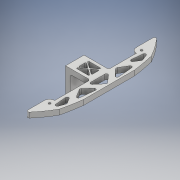
# Autodesk Inventor part: ガイド横v1
Saved by Autodesk Inventor 2018.3 (Build 223284000, 284)
## iProperties
Created: 2019-02-14
Part Number: ガイド横v1
Material: 一般
Document SubType Name: Modeling
Designer: shun2
Density: 1 g/cm^3
Appearance: 既定
Author: shun2
Autodesk Inventor part; units mm, degrees
ref_plane "YZ Plane" through (0, 0, 0) normal (1, 0, 0) x (0, 1, 0)
ref_plane "XZ Plane" through (0, 0, 0) normal (0, 1, 0) x (-1, 0, 0)
ref_plane "XY Plane" through (0, 0, 0) normal (0, 0, 1) x (1, 0, 0)
sketch "スケッチ1" plane through (0, 0, 0) normal (0, 0, 1) x (1, 0, 0)
  circle A0 centre (7, 27.638) radius 1.5
  circle A1 centre (7, 152.362) radius 1.5
  arc A2 (0, 0) -> (20.2574, 27.638) centre (-93.8083, 90) ccw
  arc A3 (20.2574, 152.362) -> (0, 180) centre (-93.8083, 90) ccw
  arc A4 (0, 152.362) -> (7, 145.362) centre (7, 152.362) ccw
  arc A5 (7, 34.638) -> (0, 27.638) centre (7, 27.638) ccw
  line L0 (7, 34.638) -> (7, 145.362)
  line L1 (0, 180) -> (0, 152.362)
  line L2 (0, 27.638) -> (0, 0)
  line L3 (25.3494, 124.4636) -> (25.3494, 55.5364)
  arc A6 (20.2574, 27.638) -> (25.3494, 55.5364) centre (-242.442, 90) ccw
  arc A7 (25.3494, 124.4636) -> (20.2574, 152.362) centre (-242.442, 90) ccw
  point P0 (7, 20.638)
  point P1 (7, 159.362)
  dimension "d2" = 3
  dimension "d11" = 27.638
  constraints: 12 point on circle, 8 centre point, 8 end point, 4 vertical, 2 coincident, 2 point on line
  measures "d2" diameter of A0
  measures "d11" vertical distance of L2.end A0.centre
extrude "押し出し1" add sketch "スケッチ1" along normal blind 7
sketch "スケッチ2" plane through (0, 0, 7) normal (0, 0, 1) x (1, 0, 0)
  line L0 (10, 80.2837) -> (10, 99.7163)
  line L1 (13.4987, 101.0407) -> (22.0846, 91.3243)
  line L2 (22.0846, 88.6757) -> (13.4987, 78.9593)
  line L3 (19.2111, 75.7008) -> (11.0046, 66.6519)
  line L4 (10.7784, 64.2673) -> (17.1291, 53.8503)
  line L5 (20.8277, 54.7016) -> (22.6836, 74.1675)
  line L6 (14.4979, 46.7358) -> (18.8075, 39.7711)
  line L7 (18.979, 38.0154) -> (16.0642, 30.2561)
  line L8 (12.2009, 30.7708) -> (10.8061, 45.4948)
  arc A0 (18.979, 38.0154) -> (18.8075, 39.7711) centre (17.1068, 38.7188) ccw
  arc A1 (11.0046, 66.6519) -> (10.7784, 64.2673) centre (12.4861, 65.3083) ccw
  arc A2 (22.0846, 88.6757) -> (22.0846, 91.3243) centre (20.5859, 90) ccw
  arc A3 (12.2009, 30.7708) -> (16.0642, 30.2561) centre (14.192, 30.9595) ccw
  arc A4 (14.4979, 46.7358) -> (10.8061, 45.4948) centre (12.7972, 45.6834) ccw
  arc A5 (17.1291, 53.8503) -> (20.8277, 54.7016) centre (18.8368, 54.8914) ccw
  arc A6 (22.6836, 74.1675) -> (19.2111, 75.7008) centre (20.6926, 74.3573) ccw
  arc A7 (10, 80.2837) -> (13.4987, 78.9593) centre (12, 80.2837) ccw
  arc A8 (13.4987, 101.0407) -> (10, 99.7163) centre (12, 99.7163) ccw
  line L9 (19.2111, 104.2992) -> (11.0046, 113.3481)
  line L10 (10.7784, 115.7327) -> (17.1291, 126.1497)
  line L11 (20.8277, 125.2984) -> (22.6836, 105.8325)
  line L12 (14.4979, 133.2642) -> (18.8075, 140.2289)
  line L13 (18.979, 141.9846) -> (16.0642, 149.7439)
  line L14 (12.2009, 149.2292) -> (10.8061, 134.5052)
  arc A9 (18.8075, 140.2289) -> (18.979, 141.9846) centre (17.1068, 141.2812) ccw
  arc A10 (10.7784, 115.7327) -> (11.0046, 113.3481) centre (12.4861, 114.6917) ccw
  arc A11 (16.0642, 149.7439) -> (12.2009, 149.2292) centre (14.192, 149.0405) ccw
  arc A12 (10.8061, 134.5052) -> (14.4979, 133.2642) centre (12.7972, 134.3166) ccw
  arc A13 (20.8277, 125.2984) -> (17.1291, 126.1497) centre (18.8368, 125.1086) ccw
  arc A14 (19.2111, 104.2992) -> (22.6836, 105.8325) centre (20.6926, 105.6427) ccw
  point P0 (0, 0)
  point P1 (10, 75)
  point P2 (10, 105)
  dimension "d17" = 30
  dimension "d18" = 2
  constraints: 30 end point, 30 point on circle, 18 tangent, 15 centre point, 8 equal radius, 4 point on line, 1 vertical
  measures "d17" distance of point (10, 75) point (10, 105)
  measures "d18" radius of A0
extrude "押し出し2" cut sketch "スケッチ2" against normal blind 7
fillet "フィレット1" radius 2 2 edges at (0, 180, 3.5) (0, 0, 3.5)
sketch "スケッチ3" plane through (0, 0, 7) normal (0, 0, 1) x (1, 0, 0)
  arc A0 (20.8277, 125.2984) -> (17.1291, 126.1497) centre (18.8368, 125.1086) ccw projected
  line L0 (17.1291, 126.1497) -> (10.7784, 115.7327) projected
  arc A1 (10.7784, 115.7327) -> (11.0046, 113.3481) centre (12.4861, 114.6917) ccw projected
  line L1 (11.0046, 113.3481) -> (19.2111, 104.2992) projected
  arc A2 (19.2111, 104.2992) -> (22.6836, 105.8325) centre (20.6926, 105.6427) ccw projected
  line L2 (22.6836, 105.8325) -> (20.8277, 125.2984) projected
  arc A3 (18.8075, 140.2289) -> (18.979, 141.9846) centre (17.1068, 141.2812) ccw projected
  line L3 (18.979, 141.9846) -> (16.0642, 149.7439) projected
  arc A4 (16.0642, 149.7439) -> (12.2009, 149.2292) centre (14.192, 149.0405) ccw projected
  line L4 (12.2009, 149.2292) -> (10.8061, 134.5052) projected
  arc A5 (10.8061, 134.5052) -> (14.4979, 133.2642) centre (12.7972, 134.3166) ccw projected
  line L5 (14.4979, 133.2642) -> (18.8075, 140.2289) projected
  arc A6 (14.4979, 46.7358) -> (10.8061, 45.4948) centre (12.7972, 45.6834) ccw projected
  line L6 (10.8061, 45.4948) -> (12.2009, 30.7708) projected
  arc A7 (12.2009, 30.7708) -> (16.0642, 30.2561) centre (14.192, 30.9595) ccw projected
  line L7 (16.0642, 30.2561) -> (18.979, 38.0154) projected
  arc A8 (18.979, 38.0154) -> (18.8075, 39.7711) centre (17.1068, 38.7188) ccw projected
  line L8 (18.8075, 39.7711) -> (14.4979, 46.7358) projected
  arc A9 (11.0046, 66.6519) -> (10.7784, 64.2673) centre (12.4861, 65.3083) ccw projected
  line L9 (10.7784, 64.2673) -> (17.1291, 53.8503) projected
  arc A10 (17.1291, 53.8503) -> (20.8277, 54.7016) centre (18.8368, 54.8914) ccw projected
  line L10 (20.8277, 54.7016) -> (22.6836, 74.1675) projected
  arc A11 (22.6836, 74.1675) -> (19.2111, 75.7008) centre (20.6926, 74.3573) ccw projected
  line L11 (19.2111, 75.7008) -> (11.0046, 66.6519) projected
  arc A12 (13.4987, 101.0407) -> (10, 99.7163) centre (12, 99.7163) ccw projected
  line L12 (10, 99.7163) -> (10, 80.2837) projected
  arc A13 (10, 80.2837) -> (13.4987, 78.9593) centre (12, 80.2837) ccw projected
  line L13 (13.4987, 78.9593) -> (22.0846, 88.6757) projected
  arc A14 (22.0846, 88.6757) -> (22.0846, 91.3243) centre (20.5859, 90) ccw projected
  line L14 (22.0846, 91.3243) -> (13.4987, 101.0407) projected
  circle A15 centre (7, 152.362) radius 1.5 projected
  circle A16 centre (7, 27.638) radius 1.5 projected
  arc A17 (0, 5.1191) -> (3.497, 3.7928) centre (2, 5.1191) ccw projected
  line L15 (0, 27.638) -> (0, 5.1191) projected
  arc A18 (7, 34.638) -> (0, 27.638) centre (7, 27.638) ccw projected
  line L16 (7, 145.362) -> (7, 34.638) projected
  arc A19 (0, 152.362) -> (7, 145.362) centre (7, 152.362) ccw projected
  line L17 (0, 174.8809) -> (0, 152.362) projected
  arc A20 (3.497, 176.2072) -> (0, 174.8809) centre (2, 174.8809) ccw projected
  arc A21 (20.2574, 152.362) -> (3.497, 176.2072) centre (-93.8083, 90) ccw projected
  arc A22 (25.3494, 124.4636) -> (20.2574, 152.362) centre (-242.442, 90) ccw projected
  line L18 (25.3494, 55.5364) -> (25.3494, 124.4636) projected
  arc A23 (20.2574, 27.638) -> (25.3494, 55.5364) centre (-242.442, 90) ccw projected
  arc A24 (3.497, 3.7928) -> (20.2574, 27.638) centre (-93.8083, 90) ccw projected
  line L19 (7, 145.362) -> (7, 34.638) projected
  line L20 (7, 82.815) -> (-26.382, 82.815)
  line L21 (-26.382, 82.815) -> (-26.382, 107.815)
  line L22 (-26.382, 107.815) -> (7, 107.815)
  line L23 (7, 107.815) -> (7, 82.815)
  point P0 (0, 0)
  dimension "d41" = 33.382
  dimension "d42" = 25
  dimension "d48" = 55.177
  constraints: 8 end point, 2 parallel, 1 horizontal, 1 perpendicular, 1 point on line
  measures "d41" distance of L21.end L22.end
  measures "d42" distance of L20.end L21.end
  measures "d48" distance from line of L20 A16.centre
extrude "押し出し3" add sketch "スケッチ3" against normal blind 7 contours L20 L21 L22 L16
sketch "スケッチ4" plane through (0, 0, 0) normal (0, 0, -1) x (-1, 0, 0)
  arc A0 (-17.1291, 126.1497) -> (-20.8277, 125.2984) centre (-18.8368, 125.1086) ccw projected
  line L0 (-17.1291, 126.1497) -> (-10.7784, 115.7327) projected
  arc A1 (-11.0046, 113.3481) -> (-10.7784, 115.7327) centre (-12.4861, 114.6917) ccw projected
  line L1 (-11.0046, 113.3481) -> (-19.2111, 104.2992) projected
  arc A2 (-22.6836, 105.8325) -> (-19.2111, 104.2992) centre (-20.6926, 105.6427) ccw projected
  line L2 (-22.6836, 105.8325) -> (-20.8277, 125.2984) projected
  arc A3 (-18.979, 141.9846) -> (-18.8075, 140.2289) centre (-17.1068, 141.2812) ccw projected
  line L3 (-18.979, 141.9846) -> (-16.0642, 149.7439) projected
  arc A4 (-12.2009, 149.2292) -> (-16.0642, 149.7439) centre (-14.192, 149.0405) ccw projected
  line L4 (-12.2009, 149.2292) -> (-10.8061, 134.5052) projected
  arc A5 (-14.4979, 133.2642) -> (-10.8061, 134.5052) centre (-12.7972, 134.3166) ccw projected
  line L5 (-14.4979, 133.2642) -> (-18.8075, 140.2289) projected
  arc A6 (-10.8061, 45.4948) -> (-14.4979, 46.7358) centre (-12.7972, 45.6834) ccw projected
  line L6 (-10.8061, 45.4948) -> (-12.2009, 30.7708) projected
  arc A7 (-16.0642, 30.2561) -> (-12.2009, 30.7708) centre (-14.192, 30.9595) ccw projected
  line L7 (-16.0642, 30.2561) -> (-18.979, 38.0154) projected
  arc A8 (-18.8075, 39.7711) -> (-18.979, 38.0154) centre (-17.1068, 38.7188) ccw projected
  line L8 (-18.8075, 39.7711) -> (-14.4979, 46.7358) projected
  arc A9 (-10.7784, 64.2673) -> (-11.0046, 66.6519) centre (-12.4861, 65.3083) ccw projected
  line L9 (-10.7784, 64.2673) -> (-17.1291, 53.8503) projected
  arc A10 (-20.8277, 54.7016) -> (-17.1291, 53.8503) centre (-18.8368, 54.8914) ccw projected
  line L10 (-20.8277, 54.7016) -> (-22.6836, 74.1675) projected
  arc A11 (-19.2111, 75.7008) -> (-22.6836, 74.1675) centre (-20.6926, 74.3573) ccw projected
  line L11 (-19.2111, 75.7008) -> (-11.0046, 66.6519) projected
  arc A12 (-10, 99.7163) -> (-13.4987, 101.0407) centre (-12, 99.7163) ccw projected
  line L12 (-10, 99.7163) -> (-10, 80.2837) projected
  arc A13 (-13.4987, 78.9593) -> (-10, 80.2837) centre (-12, 80.2837) ccw projected
  line L13 (-13.4987, 78.9593) -> (-22.0846, 88.6757) projected
  arc A14 (-22.0846, 91.3243) -> (-22.0846, 88.6757) centre (-20.5859, 90) ccw projected
  line L14 (-22.0846, 91.3243) -> (-13.4987, 101.0407) projected
  circle A15 centre (-7, 152.362) radius 1.5 projected
  circle A16 centre (-7, 27.638) radius 1.5 projected
  arc A17 (-3.497, 3.7928) -> (0, 5.1191) centre (-2, 5.1191) ccw projected
  line L15 (0, 27.638) -> (0, 5.1191) projected
  arc A18 (0, 27.638) -> (-7, 34.638) centre (-7, 27.638) ccw projected
  line L16 (-7, 145.362) -> (-7, 107.815) projected
  arc A19 (-7, 145.362) -> (0, 152.362) centre (-7, 152.362) ccw projected
  line L17 (0, 174.8809) -> (0, 152.362) projected
  arc A20 (0, 174.8809) -> (-3.497, 176.2072) centre (-2, 174.8809) ccw projected
  arc A21 (-3.497, 176.2072) -> (-20.2574, 152.362) centre (93.8083, 90) ccw projected
  arc A22 (-20.2574, 152.362) -> (-25.3494, 124.4636) centre (242.442, 90) ccw projected
  line L18 (-25.3494, 55.5364) -> (-25.3494, 124.4636) projected
  arc A23 (-25.3494, 55.5364) -> (-20.2574, 27.638) centre (242.442, 90) ccw projected
  arc A24 (-20.2574, 27.638) -> (-3.497, 3.7928) centre (93.8083, 90) ccw projected
  line L19 (26.382, 82.815) -> (20.382, 82.815)
  line L20 (20.382, 82.815) -> (20.382, 107.815)
  line L21 (20.382, 107.815) -> (26.382, 107.815)
  line L22 (26.382, 107.815) -> (26.382, 82.815)
  line L23 (-7, 82.815) -> (-7, 34.638) projected
  line L24 (-7, 82.815) -> (26.382, 82.815) projected
  line L25 (26.382, 82.815) -> (26.382, 107.815) projected
  line L26 (26.382, 107.815) -> (-7, 107.815) projected
  point P0 (0, 0)
  dimension "d37" = 6
  dimension "d43" = 0
  dimension "d44" = 0
  constraints: 8 end point, 2 parallel, 1 horizontal, 1 perpendicular
  measures "d37" distance of L20.end L21.end
  measures "d43" distance between parallel lines of L26 L21
  measures "d44" distance between parallel lines of L24 L19
extrude "押し出し4" add sketch "スケッチ4" along normal blind 31.3 contours L20 L21 L22 L19
sketch "スケッチ7" plane through (-26.382, 82.815, 7) normal (-1, 0, 0) x (0, 0, 1)
  circle A0 centre (-33.95, 12.5) radius 2.15
  line L0 (0, 0) -> (-38.3, 0) projected
  point P0 (-7, -82.815)
  dimension "d45" = 4.3
  dimension "d76" = 12.5
  constraints: 1 centre point
  measures "d45" diameter of A0
  measures "d76" distance from line of L0 A0.centre
extrude "押し出し7" cut sketch "スケッチ7" against normal blind 16.3
sketch "スケッチ8" plane through (0, 0, 0) normal (0, 0, -1) x (-1, 0, 0)
  line L0 (20.382, 82.815) -> (20.382, 107.815) projected
  line L1 (20.382, 107.815) -> (-7, 107.815) projected
  line L2 (-7, 145.362) -> (-7, 107.815) projected
  arc A0 (-7, 145.362) -> (0, 152.362) centre (-7, 152.362) ccw projected
  line L3 (0, 174.8809) -> (0, 152.362) projected
  arc A1 (0, 174.8809) -> (-3.497, 176.2072) centre (-2, 174.8809) ccw projected
  arc A2 (-3.497, 176.2072) -> (-20.2574, 152.362) centre (93.8083, 90) ccw projected
  arc A3 (-20.2574, 152.362) -> (-25.3494, 124.4636) centre (242.442, 90) ccw projected
  line L4 (-25.3494, 55.5364) -> (-25.3494, 124.4636) projected
  arc A4 (-25.3494, 55.5364) -> (-20.2574, 27.638) centre (242.442, 90) ccw projected
  arc A5 (-20.2574, 27.638) -> (-3.497, 3.7928) centre (93.8083, 90) ccw projected
  arc A6 (-3.497, 3.7928) -> (0, 5.1191) centre (-2, 5.1191) ccw projected
  line L5 (0, 27.638) -> (0, 5.1191) projected
  arc A7 (0, 27.638) -> (-7, 34.638) centre (-7, 27.638) ccw projected
  line L6 (-7, 82.815) -> (-7, 34.638) projected
  line L7 (-7, 82.815) -> (20.382, 82.815) projected
  arc A8 (-17.1291, 126.1497) -> (-20.8277, 125.2984) centre (-18.8368, 125.1086) ccw projected
  line L8 (-17.1291, 126.1497) -> (-10.7784, 115.7327) projected
  arc A9 (-11.0046, 113.3481) -> (-10.7784, 115.7327) centre (-12.4861, 114.6917) ccw projected
  line L9 (-11.0046, 113.3481) -> (-19.2111, 104.2992) projected
  arc A10 (-22.6836, 105.8325) -> (-19.2111, 104.2992) centre (-20.6926, 105.6427) ccw projected
  line L10 (-22.6836, 105.8325) -> (-20.8277, 125.2984) projected
  arc A11 (-18.979, 141.9846) -> (-18.8075, 140.2289) centre (-17.1068, 141.2812) ccw projected
  line L11 (-18.979, 141.9846) -> (-16.0642, 149.7439) projected
  arc A12 (-12.2009, 149.2292) -> (-16.0642, 149.7439) centre (-14.192, 149.0405) ccw projected
  line L12 (-12.2009, 149.2292) -> (-10.8061, 134.5052) projected
  arc A13 (-14.4979, 133.2642) -> (-10.8061, 134.5052) centre (-12.7972, 134.3166) ccw projected
  line L13 (-14.4979, 133.2642) -> (-18.8075, 140.2289) projected
  arc A14 (-10.8061, 45.4948) -> (-14.4979, 46.7358) centre (-12.7972, 45.6834) ccw projected
  line L14 (-10.8061, 45.4948) -> (-12.2009, 30.7708) projected
  arc A15 (-16.0642, 30.2561) -> (-12.2009, 30.7708) centre (-14.192, 30.9595) ccw projected
  line L15 (-16.0642, 30.2561) -> (-18.979, 38.0154) projected
  arc A16 (-18.8075, 39.7711) -> (-18.979, 38.0154) centre (-17.1068, 38.7188) ccw projected
  line L16 (-18.8075, 39.7711) -> (-14.4979, 46.7358) projected
  arc A17 (-10.7784, 64.2673) -> (-11.0046, 66.6519) centre (-12.4861, 65.3083) ccw projected
  line L17 (-10.7784, 64.2673) -> (-17.1291, 53.8503) projected
  arc A18 (-20.8277, 54.7016) -> (-17.1291, 53.8503) centre (-18.8368, 54.8914) ccw projected
  line L18 (-20.8277, 54.7016) -> (-22.6836, 74.1675) projected
  arc A19 (-19.2111, 75.7008) -> (-22.6836, 74.1675) centre (-20.6926, 74.3573) ccw projected
  line L19 (-19.2111, 75.7008) -> (-11.0046, 66.6519) projected
  arc A20 (-10, 99.7163) -> (-13.4987, 101.0407) centre (-12, 99.7163) ccw projected
  line L20 (-10, 99.7163) -> (-10, 80.2837) projected
  arc A21 (-13.4987, 78.9593) -> (-10, 80.2837) centre (-12, 80.2837) ccw projected
  line L21 (-13.4987, 78.9593) -> (-22.0846, 88.6757) projected
  arc A22 (-22.0846, 91.3243) -> (-22.0846, 88.6757) centre (-20.5859, 90) ccw projected
  line L22 (-22.0846, 91.3243) -> (-13.4987, 101.0407) projected
  circle A23 centre (-7, 152.362) radius 1.5 projected
  circle A24 centre (-7, 27.638) radius 1.5 projected
  line L23 (8.3223, 96.7373) -> (15.7997, 101.973)
  line L24 (7.7488, 96.3356) -> (16.877, 96.3356) construction
  line L25 (7.1752, 96.7373) -> (-0.3022, 101.973)
  line L26 (7.7488, 96.3356) -> (16.877, 96.3356) construction
  line L27 (0.2714, 103.7921) -> (15.2261, 103.7921)
  line L28 (8.1566, 93.9409) -> (15.634, 88.7052)
  line L29 (7.583, 94.3425) -> (16.7112, 94.3425) construction
  line L30 (7.0095, 93.9409) -> (-0.4679, 88.7052)
  line L31 (7.583, 94.3425) -> (16.7112, 94.3425) construction
  line L32 (0.1057, 86.886) -> (15.0604, 86.886)
  line L33 (9.5473, 94.5356) -> (14.9954, 90.7208)
  line L34 (8.3774, 95.3548) -> (15.0283, 95.3548) construction
  line L35 (9.5473, 96.1739) -> (14.9954, 99.9887)
  line L36 (8.3774, 95.3548) -> (15.0283, 95.3548) construction
  line L37 (16.569, 99.1696) -> (16.569, 91.54)
  line L38 (5.2076, 94.5361) -> (-0.2405, 90.7213)
  line L39 (6.3774, 95.3552) -> (13.0284, 95.3552) construction
  line L40 (-1.8141, 91.5404) -> (-1.8141, 99.1704)
  line L41 (-0.2405, 99.9895) -> (5.2077, 96.1744)
  arc A25 (0.2714, 103.7921) -> (-0.3022, 101.973) centre (0.2714, 102.7921) ccw
  arc A26 (15.7997, 101.973) -> (15.2261, 103.7921) centre (15.2261, 102.7921) ccw
  arc A27 (7.1752, 96.7373) -> (8.3223, 96.7373) centre (7.7488, 97.5564) ccw
  arc A28 (15.0604, 86.886) -> (15.634, 88.7052) centre (15.0604, 87.886) ccw
  arc A29 (-0.4679, 88.7052) -> (0.1057, 86.886) centre (0.1057, 87.886) ccw
  arc A30 (8.1566, 93.9409) -> (7.0095, 93.9409) centre (7.583, 93.1217) ccw
  arc A31 (16.569, 99.1696) -> (14.9954, 99.9887) centre (15.569, 99.1696) ccw
  arc A32 (14.9954, 90.7208) -> (16.569, 91.54) centre (15.569, 91.54) ccw
  arc A33 (9.5473, 96.1739) -> (9.5473, 94.5356) centre (10.1209, 95.3548) ccw
  arc A34 (5.2076, 94.5361) -> (5.2077, 96.1744) centre (4.6341, 95.3552) ccw
  arc A35 (-1.8141, 91.5404) -> (-0.2405, 90.7213) centre (-0.8141, 91.5404) ccw
  arc A36 (-0.2405, 99.9895) -> (-1.8141, 99.1704) centre (-0.8141, 99.1704) ccw
  point P0 (0, 0)
  point P1 (18.3977, 103.7921)
  point P2 (18.232, 86.886)
  point P3 (-3.0659, 86.886)
  point P4 (16.569, 89.619)
  point P5 (16.569, 101.0905)
  point P6 (-1.8141, 89.6194)
  dimension "d56" = 2
  dimension "d57" = 2
  dimension "d58" = 13
  dimension "d59" = 35
  dimension "d60" = 145
  dimension "d61" = 13
  dimension "d62" = 35
  dimension "d63" = 13
  dimension "d64" = 145
  dimension "d65" = 10
  dimension "d66" = 35
  dimension "d67" = 10
  dimension "d68" = 35
  dimension "d69" = 10
  dimension "d70" = 145
  dimension "d71" = 1
  dimension "d72" = 8.7254
  dimension "d73" = 7.63
  dimension "d77" = 8.725
  constraints: 38 end point, 24 point on circle, 24 tangent, 20 point on line, 12 centre point, 11 equal radius, 8 horizontal, 7 equal length, 1 parallel, 1 vertical
  measures "d56" distance of L29.start L24.start
  measures "d57" distance of L39.start L34.start
  measures "d58" distance of L24.start point (18.398, 103.792)
  measures "d59" angle of L24 L23
  measures "d60" angle of L26 L25
  measures "d61" distance of L29.start point (18.232, 86.886)
  measures "d62" angle of L28 L29
  measures "d63" distance of L29.start point (-3.066, 86.886)
  measures "d64" angle of L30 L31
  measures "d65" distance of L34.start point (16.569, 89.619)
  measures "d66" angle of L33 L34
  measures "d67" distance of L34.start point (16.569, 101.091)
  measures "d68" angle of L36 L35
  measures "d69" distance of L39.start point (-1.814, 89.619)
  measures "d70" angle of L38 L39
  measures "d71" radius of A25
  measures "d72" distance from line of L7 L40.start
  measures "d73" distance of L40.start L40.end
  measures "d77" distance from line of L7 L37.end
extrude "押し出し8" cut sketch "スケッチ8" against normal blind 16.3 contours A27 L25 A25 L27 A26 L23 | L28 A28 L32 A29 L30 A30 | A33 L35 A31 L37 A32 L33 | L38 A35 L40 A36 L41 A34
chamfer "面取り1" distance 2 angle 45 5 edges at (-20.382, 95.315, 0) (7, 107.815, 3.5) (7, 82.815, 3.5) (-23.382, 82.815, -31.3) (-23.382, 107.815, -31.3)
